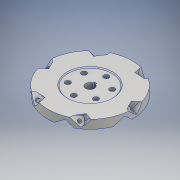
# Autodesk Inventor part: CheekPlate
Saved by Autodesk Inventor 2018 (Build 220112000, 112)
## iProperties
Created: 2017-09-05
Part Number: CheekPlate
Material: Aluminum 6061
Document SubType Name: Modeling
Designer: P136265
Density: 2.7 g/cm^3
Appearance: Aluminum - Flat
Mass: 1196.04 g
Surface Area: 792.054 cm^2
Volume: 442.977 cm^3
Author: P136265
Autodesk Inventor part; units mm, degrees
ref_plane "Work Plane1" through (0, 0, 50) normal (0, 0, 1) x (1, 0, 0)
sketch "Sketch1" plane through (0, 0, 50) normal (0, 0, 1) x (1, 0, 0)
  circle A0 centre (0, 0) radius 97
  dimension "d1" = 194
  constraints: 1 centre point, 1 coincident
  measures "d1" diameter of A0
extrude "Extrusion1" add sketch "Sketch1" along normal mid plane 20
ref_plane "Work Plane8" through (43.4971, -89.2355, 43.4971) normal (0.7071068, 0, 0.7071068) x (0, 1, 0)
sketch "Sketch3" plane through (43.4971, -89.2355, 43.4971) normal (0.7071068, 0, 0.7071068) x (0, 1, 0)
  point P0 (89.2355, 0)
ref_plane "Work Plane9" through (0, 0, 0) normal (0.7071068, 0, -0.7071068) x (0, 1, 0)
sketch "Sketch4" plane through (0, 0, 0) normal (0.7071068, 0, -0.7071068) x (0, 1, 0)
  spline S0 degree 3 poles (-89.2355, -61.5142) (-90.3927, -58.6064) (-92.539, -52.544) (-94.7745, -44.4386) (-96.6571, -36.0105) (-97.8745, -29.0401) (-99.0232, -20.1209) (-99.6396, -12.8528) (-100.0257, -3.6842) (-100.0257, 3.6842) (-99.6396, 12.8528) (-99.0232, 20.1209) (-97.8745, 29.0401) (-96.6571, 36.0105) (-94.7745, 44.4386) (-92.539, 52.544) (-90.3927, 58.6064) (-89.2355, 61.5142) knots 4.04016 4.04016 4.04016 4.04016 4.152198 4.264236 4.320255 4.432293 4.488313 4.600351 4.65637 4.768408 4.824427 4.936465 4.992485 5.104523 5.160542 5.27258 5.384618 5.384618 5.384618 5.384618 construction
  line L0 (-89.2355, 61.5142) -> (-60.7645, 61.5142) construction
  line L1 (-89.2355, -61.5142) -> (-60.7645, -61.5142) construction
  line L2 (-75, 61.5142) -> (-75, 62.5142) construction
  line L3 (-75, 62.5142) -> (-93.2355, 62.5142)
  line L4 (-93.2355, 62.5142) -> (-96.2355, 62.5142)
  line L5 (-75, -61.5142) -> (-75, -62.5142) construction
  line L6 (-75, -62.5142) -> (-89.2355, -62.5142)
  line L7 (-89.2355, -62.5142) -> (-96.2355, -62.5142)
  line L8 (-75, 62.5142) -> (-75, -62.5142)
  line L9 (-75, 0) -> (-107, 0) construction
  arc A0 (-107, 0) -> (-96.2355, -62.5142) centre (79.9064, 0) ccw
  arc A1 (-96.2355, 62.5142) -> (-107, 0) centre (79.9064, 0) ccw
  point P0 (0, 0)
  dimension "d5" = 1
  dimension "d7" = 1
  dimension "d11" = 186.9064
  dimension "d70" = 7
  constraints: 16 end point, 4 point on circle, 3 midpoint, 2 centre point, 2 perpendicular, 2 point on line, 2 vertical, 1 horizontal, 1 parallel, 1 other
  measures "d5" distance of L2.start L2.end
  measures "d7" distance of L5.start L5.end
  measures "d11" radius of A1
  measures "d70" horizontal distance of L7.end L1.start
revolve "Revolution1" cut sketch "Sketch4" angle 360 about axis through (44.2042, -75, 44.2042) along (-0.7071068, 0, -0.7071068)
ref_plane "Work Plane10" through (71.7613, -75, 71.7613) normal (0.7071068, 0, 0.7071068) x (-0.2977096, -0.9070491, 0.2977096)
sketch "Sketch5" plane through (71.7613, -75, 71.7613) normal (0.7071068, 0, 0.7071068) x (-0.2977096, -0.9070491, 0.2977096)
  circle A0 centre (0, 0) radius 3.5 construction
  arc A1 (0, 10) -> (-10, 0) centre (0, 0) ccw
  line L0 (-10, -10) -> (-10, 0)
  line L1 (-10, -10) -> (0, -10)
  line L2 (10, -10) -> (0, -10)
  line L3 (10, -10) -> (20, -10)
  line L4 (20, -10) -> (20, 10)
  line L5 (20, 10) -> (0, 10)
  point P0 (-68.0287, -31.5769)
  dimension "d14" = 20
  dimension "d68" = 10
  dimension "d69" = 10
  dimension "d71" = 10
  dimension "d73" = 30
  constraints: 12 end point, 3 tangent, 2 horizontal, 2 point on circle, 1 centre point, 1 coincident, 1 parallel, 1 perpendicular, 1 vertical
  measures "d14" diameter of A1
  measures "d68" distance from line of L0 A0.centre
  measures "d69" distance from line of A0.centre L1
  measures "d71" distance of L2.start L1.end
  measures "d73" distance between parallel lines of L4 L0
extrude "Extrusion2" cut sketch "Sketch5" against normal blind 30
sketch "Sketch6" plane through (50.5481, -75, 50.5481) normal (0.7071068, 0, 0.7071068) x (0.6413805, -0.421025, -0.6413805)
  circle A0 centre (0, 0) radius 4 construction
  circle A1 centre (0, 0) radius 4.125
  point P0 (-31.5769, 68.0287)
  dimension "d17" = 8.25
  constraints: 1 centre point, 1 coincident
  measures "d17" diameter of A1
extrude "Extrusion3" cut sketch "Sketch6" against normal blind 10
pattern_circular "Circular Pattern1" count 6 over 360 about axis through (0, 0, 50) along (0, 0, 1) of "Extrusion2"
pattern_circular "Circular Pattern2" count 6 over 360 about axis through (0, 0, 50) along (0, 0, 1) of "Extrusion3"
pattern_circular "Circular Pattern3" count 6 over 360 about axis through (0, 0, 50) along (0, 0, 1) of "Revolution1"
sketch "Sketch7" plane through (0, 0, 60) normal (0, 0, 1) x (1, 0, 0)
  line L0 (55.5445, 79.5224) -> (48.7739, 75.6134) construction
  circle A0 centre (0, 0) radius 68.4904 construction
  line L1 (-41.0962, 87.8641) -> (-41.0962, 80.0462) construction
  ellipse E0 centre (34.9519, 89.4615) end of major axis (42.023, 77.2141) minor radius 10 (23.7892, 94.0376) -> (24.1195, 90.0828) ccw construction
  line L2 (-47.967, 84.31) -> (23.7892, 94.0376) construction
  arc A1 (-47.967, 84.31) -> (23.7892, 94.0376) centre (-14.7404, 108.7325) ccw
  arc A2 (23.7892, 94.0376) -> (-47.967, 84.31) centre (-9.4374, 69.6151) ccw
  point P0 (50.298, 76.4933)
  point P1 (29.7015, 61.7152)
  point P2 (-41.0962, 81.806)
  point P3 (-38.5962, 56.5798)
  point P4 (46.1299, 85.329)
  point P5 (22.9886, 66.1301)
  point P6 (-41.0962, 80.0462)
  point P7 (37.7195, 76.2474)
  constraints: 5 point on circle, 3 centre point, 2 end point, 1 coincident, 1 symmetric about line, 1 tangent, 4 other
extrude "Extrusion4" [suppressed]
pattern_circular "Circular Pattern4" [suppressed]
fillet "Fillet1" [suppressed]
pattern_circular "Circular Pattern5" [suppressed]
sketch "Sketch8" plane through (0, 0, 60) normal (0, 0, 1) x (1, 0, 0)
  circle A0 centre (0, 0) radius 52.5
  dimension "d39" = 105
  constraints: 1 centre point, 1 coincident
  measures "d39" diameter of A0
extrude "Extrusion5" cut sketch "Sketch8" against normal blind 2
sketch "Sketch9" plane through (0, 0, 40) normal (0, 0, -1) x (-1, 0, 0)
  circle A0 centre (0, 0) radius 52.5
  dimension "d42" = 105
  constraints: 1 centre point, 1 coincident
  measures "d42" diameter of A0
extrude "Extrusion6" [suppressed]
chamfer "Chamfer1" distance 2 angle 45 1 edges at (-52.5, 0, 58)
sketch "Sketch10" plane through (0, 0, 58) normal (0, 0, 1) x (1, 0, 0)
  arc A0 (-3, 9.5394) -> (3, 9.5394) centre (0, 0) ccw
  line L0 (0, 0) -> (0, 15) construction
  line L1 (3, 9.5394) -> (3, 12.6)
  line L2 (-3, 9.5394) -> (-3, 12.6)
  line L3 (-2.8, 12.8) -> (2.8, 12.8)
  arc A1 (-2.8, 12.8) -> (-3, 12.6) centre (-2.8, 12.6) ccw
  arc A2 (3, 12.6) -> (2.8, 12.8) centre (2.8, 12.6) ccw
  point P0 (3, 12.8)
  point P1 (-3, 12.8)
  dimension "d48" = 20
  dimension "d49" = 15
  dimension "d50" = 3
  dimension "d51" = 3
  dimension "d52" = 12.8
  dimension "d93" = 0.2
  constraints: 8 end point, 6 point on circle, 4 point on line, 4 tangent, 3 centre point, 2 parallel, 1 coincident, 1 equal radius, 1 horizontal, 1 vertical
  measures "d48" diameter of A0
  measures "d49" distance of L0.start L0.end
  measures "d50" distance between parallel lines of L0 L1
  measures "d51" distance between parallel lines of L0 L2
  measures "d52" distance from line of point (0, 0) L3
  measures "d93" radius of A1
extrude "Extrusion7" cut sketch "Sketch10" against normal up to next
sketch "Sketch11" plane through (0, 0, 58) normal (0, 0, 1) x (1, 0, 0)
  arc A0 (-3, 9.5394) -> (3, 9.5394) centre (0, 0) ccw construction
  circle A1 centre (0, 0) radius 37.5 construction
  circle A2 centre (0, 37.5) radius 3.25
  dimension "d55" = 75
  dimension "d56" = 6.5
  constraints: 2 vertical alignment, 1 centre point, 1 coincident, 2 other
  measures "d56" diameter of A2
extrude "Extrusion8" cut sketch "Sketch11" against normal up to next
pattern_circular "Circular Pattern6" count 6 over 360 about axis through (0, 0, 59) along (0, 0, 1) of "Extrusion8"
sketch "Sketch12" plane through (0, 0, 58) normal (0, 0, 1) x (1, 0, 0)
  circle A0 centre (0, 37.5) radius 3.25 construction
  circle A1 centre (0, 37.5) radius 6
  point P0 (0, 0)
  dimension "d62" = 12
  constraints: 1 centre point, 1 coincident
  measures "d62" diameter of A1
extrude "Extrusion9" cut sketch "Sketch12" against normal blind 6
pattern_circular "Circular Pattern7" count 6 over 360 about axis through (0, 0, 59) along (0, 0, 1) of "Extrusion9"
fillet "Fillet2" radius 3 1 edges at (40.4591, 59.2546, 57.322)
pattern_circular "Circular Pattern8" count 6 over 360 about axis through (0, 0, 58) along (0, 0, -1) of "Fillet2"
body "Solid1"
